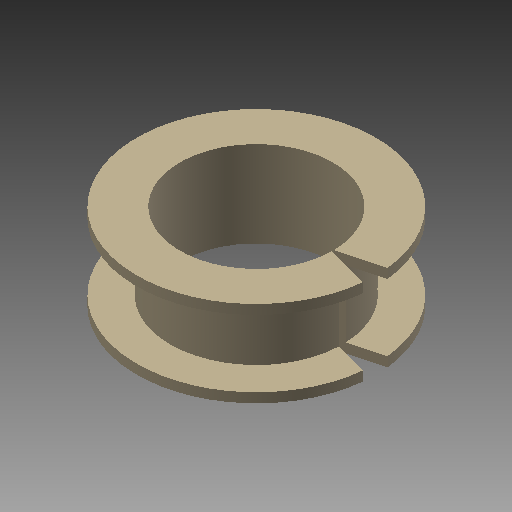
# Autodesk Inventor part: 314-14
Saved by Autodesk Inventor 2019 (Build 230136000, 136)
## iProperties
Company: Autodesk Inc.
Created: 2007-10-25
Part Number: 314-14
Document SubType Name: Modeling
Designer: Autodesk Inc.
Density: 1.13 g/cm^3
Mass: 0.132414 g
Surface Area: 5.13448 cm^2
Volume: 0.117181 cm^3
Material: Nylon-6/6
Description: SPLIT BUSHING 8 MM
Appearance: Beige
Component Category: Fasteners
Author: Inventor
Autodesk Inventor part; units mm, degrees
ref_plane "YZ Plane" through (0, 0, 0) normal (1, 0, 0) x (0, 1, 0)
ref_plane "XZ Plane" through (0, 0, 0) normal (0, 1, 0) x (-1, 0, 0)
ref_plane "XY Plane" through (0, 0, 0) normal (0, 0, 1) x (1, 0, 0)
sketch "Sketch1" plane through (0, 0, 0) normal (0, 0, 1) x (1, 0, 0)
  line L0 (0, -3.15) -> (0, 3.15) projected
  line L1 (-1.25, 0) -> (7.5, 0) projected
  line L2 (4, -2.25) -> (4, 2.25)
  line L3 (4, 2.25) -> (6.25, 2.25)
  line L4 (6.25, 2.25) -> (6.25, 1.75)
  line L5 (6.25, 1.75) -> (4.5, 1.75)
  line L6 (4.5, 1.75) -> (4.5, -1.75)
  line L7 (4.5, -1.75) -> (6.25, -1.75)
  line L8 (6.25, -1.75) -> (6.25, -2.25)
  line L9 (6.25, -2.25) -> (4, -2.25)
  point P0 (0, 0)
  point P1 (4.5, 0)
  dimension "d0" = 8
  dimension "d1" = 9
  dimension "d2" = 12.5
  dimension "d3" = 0.5
  dimension "d4" = 3.5
  dimension "d5" = 0.5
  constraints: 16 end point, 6 parallel, 2 perpendicular, 1 collinear, 1 midpoint, 1 point on line
  measures "d0" diameter of L2 L0
  measures "d1" diameter of L6 L0
  measures "d2" diameter of L4 L0
  measures "d3" distance between parallel lines of L7 L9
  measures "d4" distance between parallel lines of L5 L7
  measures "d5" distance between parallel lines of L3 L5
revolve "Revolution1" add sketch "Sketch1" angle 360 about axis through (0, -10, 0) along (0, 1, 0)
sketch "Sketch2" plane through (0, 2.25, 0) normal (0, 1, 0) x (1, 0, 0)
  circle A0 centre (0, 0) radius 6.25 projected
  circle A1 centre (0, 0) radius 4 projected
  line L0 (-8.75, 0) -> (8.75, 0) projected
  line L1 (0, 8.75) -> (0, -8.75) projected
  line L2 (3.9996, -0.0535) -> (6.2164, -0.6475)
  line L3 (3.9996, 0.0535) -> (6.2164, 0.6475)
  arc A2 (3.9996, -0.0535) -> (3.9996, 0.0535) centre (0, 0) ccw
  arc A3 (6.2164, -0.6475) -> (6.2164, 0.6475) centre (0, 0) ccw
  dimension "d8" = 15
  dimension "d9" = 30
  dimension "d10" = 2.2167
  dimension "d11" = 2.2167
  constraints: 8 point on circle, 4 end point, 2 centre point, 2 coincident
  measures "d8" angle of L2 L0
  measures "d9" angle of L3 L2
  measures "d10" horizontal distance of L2.start L2.end
  measures "d11" horizontal distance of L3.start L3.end
extrude "Extrusion1" cut sketch "Sketch2" against normal through all contours L0 A1 L3 A0 | A0 L2 A1 L0
body "Solid1"
